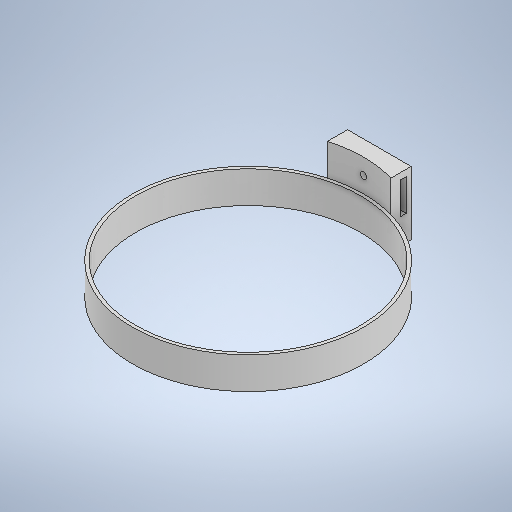
# Autodesk Inventor part: PVC_Mount
Saved by Autodesk Inventor 2025 (Build 290162010, 162A)
## iProperties
Created: 2024-06-25
Part Number: PVC_Mount
Material: Generic
Document SubType Name: Modeling
Designer: vncnt
Density: 1 g/cm^3
Appearance: Default
Author: vncnt
Autodesk Inventor part; units mm, degrees
ref_plane "YZ Plane" through (0, 0, 0) normal (1, 0, 0) x (0, 1, 0)
ref_plane "XZ Plane" through (0, 0, 0) normal (0, 1, 0) x (-1, 0, 0)
ref_plane "XY Plane" through (0, 0, 0) normal (0, 0, 1) x (1, 0, 0)
sketch "Sketch1" plane through (0, 0, 0) normal (0, 1, 0) x (-1, 0, 0)
  circle A0 centre (0, 0) radius 44.831
  circle A1 centre (0, 0) radius 46.101
  dimension "d0" = 89.662
  dimension "d1" = 92.202
  constraints: 2 centre point, 2 coincident
  measures "d0" diameter of A0
  measures "d1" diameter of A1
extrude "Extrusion1" add sketch "Sketch1" along normal blind 12.7
sketch "Sketch2" plane through (0, 12.7, 0) normal (0, 1, 0) x (1, 0, 0)
  line L0 (-12.7, 44.2878) -> (-12.7, 52.3875)
  line L1 (-12.7, 52.3875) -> (12.7, 52.3875)
  line L2 (12.7, 52.3875) -> (12.7, 44.2878)
  line L3 (12.7, 44.2878) -> (-12.7, 52.3875) construction
  line L4 (-12.7, 44.2878) -> (12.7, 52.3875) construction
  arc A0 (12.7, 44.2878) -> (-12.7, 44.2878) centre (0, 0.7181) ccw
  point P0 (0, 0)
  point P1 (0, 48.3376)
  dimension "d8" = 25.4
  dimension "d9" = 8.0997
  constraints: 10 end point, 2 midpoint, 2 point on circle, 1 centre point, 1 parallel
  measures "d8" distance of L0.end L1.end
  measures "d9" distance of L1.end L2.end
extrude "Extrusion2" add sketch "Sketch2" along normal blind 12.7 and the other way blind 12.7
sketch "Sketch3" plane through (12.7, 25.4, -52.3875) normal (0, 0, -1) x (-1, 0, 0)
  line L0 (0, -25.4) -> (0, 0) projected
  line L1 (0, 0) -> (25.4, 0) projected
  point P0 (12.7, -25.4)
  point P1 (12.7, -6.35)
  dimension "d10" = 12.7
  dimension "d11" = 6.35
  measures "d10" distance from line of L0 point (12.7, -6.35)
  measures "d11" distance from line of L1 point (12.7, -6.35)
hole "Hole1" at (0, 19.05, -52.3875) direction (0, 0, 1) diameter 2.54 depth 10.979
sketch "Sketch4" plane through (12.7, 0, -52.3875) normal (1, 0, 0) x (0, 0, -1)
  line L0 (-4.445, 22.86) -> (-1.905, 22.86)
  line L1 (-1.905, 22.86) -> (-1.905, 10.16)
  line L2 (-1.905, 10.16) -> (-4.445, 10.16)
  line L3 (-4.445, 10.16) -> (-4.445, 22.86)
  line L4 (-4.445, 22.86) -> (-1.905, 10.16) construction
  line L5 (-1.905, 22.86) -> (-4.445, 10.16) construction
  line L6 (-8.0997, 25.4) -> (0, 25.4) projected
  point P0 (-52.3875, 0)
  point P1 (-3.175, 16.51)
  dimension "d19" = 2.54
  dimension "d20" = 12.7
  dimension "d21" = 8.89
  constraints: 12 end point, 2 midpoint, 2 parallel, 1 horizontal, 1 perpendicular
  measures "d19" distance of L1.end L2.end
  measures "d20" distance of L0.end L1.end
  measures "d21" distance from line of L6 point (-3.175, 16.51)
extrude "Extrusion3" cut sketch "Sketch4" against normal through all
body "Solid1"
